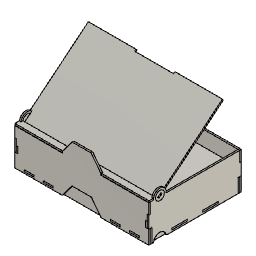
boite_h120_ep5_v2 (Autodesk Fusion 360 design; units mm, degrees)
Autodesk Fusion 360 part; units mm, degrees
note: some values were not read from the file. Set by a fixed rule: which sketch regions a step uses.
sketch "Esquisse1" plane through (0, 0, 0) normal (0, 1, 0) x (-1, 0, 0)
  line L0 (0, 0) -> (420, 0)
  line L1 (420, 0) -> (420, 120)
  line L2 (420, 120) -> (0, 120)
  line L3 (0, 120) -> (0, 0)
  line L4 (210, 0) -> (210, 120) construction
  line L5 (210, 40) -> (180, 40)
  line L6 (180, 40) -> (150, 0)
  line L7 (240, 40) -> (270, 0)
  line L8 (210, 40) -> (240, 40)
  line L9 (180, 160) -> (150, 120)
  line L10 (210, 160) -> (180, 160)
  line L11 (210, 160) -> (240, 160)
  line L12 (240, 160) -> (270, 120)
  line L13 (150, 5) -> (120, 5)
  line L14 (120, 5) -> (120, 10)
  line L15 (120, 10) -> (150, 10)
  line L16 (150, 10) -> (150, 5)
  line L17 (120, 5) -> (90, 5)
  line L18 (90, 5) -> (90, 10)
  line L19 (90, 10) -> (120, 10)
  line L20 (120, 10) -> (120, 5)
  line L21 (90, 5) -> (60, 5)
  line L22 (60, 5) -> (60, 10)
  line L23 (60, 10) -> (90, 10)
  line L24 (90, 10) -> (90, 5)
  line L25 (60, 5) -> (30, 5)
  line L26 (30, 5) -> (30, 10)
  line L27 (30, 10) -> (60, 10)
  line L28 (60, 10) -> (60, 5)
  line L29 (30, 5) -> (0, 5)
  line L30 (0, 5) -> (0, 10)
  line L31 (0, 10) -> (30, 10)
  line L32 (30, 10) -> (30, 5)
  line L33 (330, 5) -> (330, 10)
  line L34 (360, 10) -> (330, 10)
  line L35 (360, 5) -> (360, 10)
  line L36 (300, 10) -> (300, 5)
  line L37 (270, 5) -> (300, 5)
  line L38 (330, 5) -> (360, 5)
  line L39 (390, 5) -> (390, 10)
  line L40 (330, 10) -> (330, 5)
  line L41 (360, 10) -> (360, 5)
  line L42 (300, 5) -> (330, 5)
  line L43 (360, 5) -> (390, 5)
  line L44 (420, 5) -> (420, 10)
  line L45 (270, 10) -> (270, 5)
  line L46 (390, 10) -> (390, 5)
  line L47 (300, 10) -> (270, 10)
  line L48 (330, 10) -> (300, 10)
  line L49 (420, 10) -> (390, 10)
  line L50 (300, 5) -> (300, 10)
  line L51 (390, 10) -> (360, 10)
  line L52 (390, 5) -> (420, 5)
  line L53 (0, 5) -> (10, 5)
  line L54 (10, 5) -> (10, 43.3333)
  line L55 (10, 43.3333) -> (0, 43.3333)
  line L56 (0, 43.3333) -> (0, 5)
  line L57 (0, 43.3333) -> (10, 43.3333)
  line L58 (10, 81.6667) -> (0, 81.6667)
  line L59 (10, 43.3333) -> (10, 81.6667)
  line L60 (0, 81.6667) -> (10, 81.6667)
  line L61 (10, 120) -> (0, 120)
  line L62 (10, 81.6667) -> (10, 120)
  line L63 (410, 120) -> (420, 120)
  line L64 (420, 43.3333) -> (410, 43.3333)
  line L65 (410, 43.3333) -> (420, 43.3333)
  line L66 (410, 5) -> (410, 43.3333)
  line L67 (410, 81.6667) -> (410, 120)
  line L68 (420, 43.3333) -> (420, 5)
  line L69 (420, 5) -> (410, 5)
  line L70 (410, 81.6667) -> (420, 81.6667)
  line L71 (420, 81.6667) -> (410, 81.6667)
  line L72 (410, 43.3333) -> (410, 81.6667)
  line L73 (420, 5) -> (420, 10)
  line L74 (5, 43.3333) -> (5, 81.6667)
  line L75 (10, 62.5) -> (0, 62.5)
  line L76 (415, 81.6667) -> (415, 43.3333)
  line L77 (410, 62.5) -> (420, 62.5)
  line L78 (270, 120) -> (400, 120)
  line L79 (400, 120) -> (400, 115)
  line L80 (400, 115) -> (270, 115)
  line L81 (270, 115) -> (270, 120)
  line L82 (150, 120) -> (0, 120)
  line L83 (0, 120) -> (0, 115)
  line L84 (0, 115) -> (150, 115)
  line L85 (150, 115) -> (150, 120)
  line L86 (270, 115) -> (420, 115)
  line L87 (179.7, 40.6) -> (149.25, 0)
  line L88 (210, 40.6) -> (179.7, 40.6)
  line L89 (210, 40.6) -> (240.3, 40.6)
  line L90 (240.3, 40.6) -> (270.75, 0)
  point P0 (420, 120)
  dimension "d1" = 420
  dimension "d2" = 120
  dimension "d4" = 60
  dimension "d5" = 40
  dimension "d6" = 30
  dimension "d9" = 0
  dimension "d10" = 120
  dimension "d11" = 30
  dimension "d12" = 5
  dimension "d13" = 5
  dimension "d14" = 150
  dimension "d17" = -120
  dimension "d18" = 0
  dimension "d19" = 10
  dimension "d20" = 115
  dimension "d21" = 38.3333
  dimension "d24" = 0
  dimension "d25" = 76.6667
  dimension "d72" = 5
  dimension "d73" = 5
  constraint horizontal L0
  constraint vertical L1
  constraint horizontal L2
  constraint vertical L3
  constraint coincident L0.start L3.end
  constraint midpoint L0 L4.start
  constraint midpoint L2 L4.end
  constraint coincident L4 L5.start
  constraint perpendicular L4 L5
  constraint coincident L0 L6.end
  constraint symmetric L4 L5.start L8.start
  constraint symmetric L4 L5.end L7.start
  constraint symmetric L4 L6.end L7.end
  constraint horizontal L13
  constraint vertical L14
  constraint horizontal L15
  constraint vertical L16
  constraint coincident L6.end L16
  constraint symmetric L4 L13.start L37.start
  constraint symmetric L4 L13.end L36.end
  constraint symmetric L4 L14.end L36.start
  constraint symmetric L4 L15.end L45.start
  constraint symmetric L4 L17.end L33.start
  constraint symmetric L4 L18.end L33.end
  constraint symmetric L4 L21.end L35.start
  constraint symmetric L4 L22.end L34.start
  constraint symmetric L4 L25.end L39.start
  constraint symmetric L4 L26.end L39.end
  constraint symmetric L4 L29.end L44.start
  constraint symmetric L4 L30.end L44.end
  constraint horizontal L53
  constraint vertical L54
  constraint horizontal L55
  constraint vertical L56
  constraint symmetric L2.end L4 P0
  constraint symmetric L4 L53.end L66.start
  constraint symmetric L4 L54.end L64.end
  constraint symmetric L4 L55.end L64.start
  constraint symmetric L4 L58.start L67.start
  constraint symmetric L4 L58.end L70.end
  constraint symmetric L4 L61.start L63.start
  constraint symmetric L4 L2.end P0
  constraint midpoint L57 L74.start
  constraint midpoint L60 L74.end
  constraint midpoint L59 L75.start
  constraint coincident L3 L75.end
  constraint perpendicular L3 L75
  constraint midpoint L70 L76.start
  constraint midpoint L64 L76.end
  constraint midpoint L72 L77.start
  constraint coincident L1 L77.end
  constraint perpendicular L1 L77
  constraint horizontal L78
  constraint vertical L79
  constraint horizontal L80
  constraint vertical L81
  constraint horizontal L82
  constraint vertical L83
  constraint horizontal L84
  constraint vertical L85
  constraint coincident L1 L86.end
  constraint perpendicular L1 L86
  constraint coincident L0 L90.end
  constraint coincident L0 L87.end
  measures "d1" distance of L0.start L0.end
  measures "d2" distance of L0.start L2.end
  measures "d4" distance of L4.start L6.end
  measures "d5" distance of L0 L5
  measures "d6" distance of L5.start L5.end
  measures "d11" distance of L13.start L13.end
  measures "d12" distance of L13.start L15.end
  measures "d13" distance of L0 L13
  measures "d14" distance of L0.start L6.end
  measures "d19" distance of L54.end L55.end
  measures "d20" distance of L2 L29
  measures "d21" distance of L53 L55
  measures "d72" distance of L12.end L80.end
  measures "d73" distance of L9.end L84.end
extrude "Extrusion1" add sketch "Esquisse1" along normal blind 5 contours L0 L1 L2 L3 L13 L15 L16 L17 L19 L21 L23 L25 L27 L29 L31 L34 L37 L38 L42 L43 L45 L47 L48 L49 L51 L52 L53 L54 L59 L62 L66 L67 L69 L72 L80 L81 L84 L85 L86 L87 L88 L89 L90 | L3 L29 L30 L31 L53 L54 L56 | L3 L31 L54 L55 L56 L57 | L26 L29 L31 L32 L54 | L18 L21 L22 L23 L24 L28 | L3 L58 L60 L62 L84 | L58 L59 L60 L74 L75 | L1 L44 L49 L52 L66 L68 L69 L73 | L13 L14 L15 L16 L20 | L1 L49 L64 L65 L66 L68 | L39 L46 L49 L52 L66 | L33 L34 L35 L38 L40 L41 | L2 L9 L10 L11 L12 | L1 L67 L70 L71 L86 | L70 L71 L72 L76 L77 | L36 L37 L45 L47 L50 makes body 1
sketch "Esquisse2" plane through (0, 5, 0) normal (0, 1, 0) x (-1, 0, 0)
  line L0 (420, 0) -> (0, 0)
  line L1 (0, 0) -> (0, 62.5)
  line L2 (0, 62.5) -> (420, 62.5)
  line L3 (420, 62.5) -> (420, 0)
  line L4 (0, 10) -> (30, 10)
  line L5 (30, 10) -> (30, 5)
  line L6 (30, 5) -> (0, 5)
  line L7 (0, 5) -> (0, 10)
  line L8 (210, 62.5) -> (210, 0) construction
  line L9 (30, 10) -> (60, 10)
  line L10 (60, 5) -> (30, 5)
  line L11 (30, 5) -> (30, 10)
  line L12 (60, 10) -> (60, 5)
  line L13 (60, 10) -> (90, 10)
  line L14 (90, 5) -> (60, 5)
  line L15 (60, 5) -> (60, 10)
  line L16 (90, 10) -> (90, 5)
  line L17 (90, 10) -> (120, 10)
  line L18 (120, 5) -> (90, 5)
  line L19 (90, 5) -> (90, 10)
  line L20 (120, 10) -> (120, 5)
  line L21 (120, 10) -> (150, 10)
  line L22 (150, 5) -> (120, 5)
  line L23 (120, 5) -> (120, 10)
  line L24 (150, 10) -> (150, 5)
  line L25 (0, 62.5) -> (10, 62.5)
  line L26 (10, 62.5) -> (10, 43.3333)
  line L27 (10, 43.3333) -> (0, 43.3333)
  line L28 (0, 43.3333) -> (0, 62.5)
  line L29 (270, 10) -> (270, 5)
  line L30 (420, 62.5) -> (410, 62.5)
  line L31 (300, 10) -> (270, 10)
  line L32 (410, 43.3333) -> (420, 43.3333)
  line L33 (300, 5) -> (300, 10)
  line L34 (300, 5) -> (330, 5)
  line L35 (360, 5) -> (360, 10)
  line L36 (390, 5) -> (420, 5)
  line L37 (410, 62.5) -> (410, 43.3333)
  line L38 (270, 5) -> (300, 5)
  line L39 (420, 5) -> (420, 10)
  line L40 (330, 5) -> (330, 10)
  line L41 (390, 10) -> (360, 10)
  line L42 (420, 43.3333) -> (420, 62.5)
  line L43 (300, 10) -> (300, 5)
  line L44 (360, 10) -> (330, 10)
  line L45 (330, 10) -> (330, 5)
  line L46 (360, 10) -> (360, 5)
  line L47 (390, 5) -> (390, 10)
  line L48 (330, 10) -> (300, 10)
  line L49 (420, 0) -> (420, 62.5)
  line L50 (390, 10) -> (390, 5)
  line L51 (360, 5) -> (390, 5)
  line L52 (420, 10) -> (390, 10)
  line L53 (330, 5) -> (360, 5)
  line L54 (90, 10) -> (120, 10)
  line L55 (120, 10) -> (120, 5)
  line L56 (120, 5) -> (90, 5)
  line L57 (90, 5) -> (90, 10)
  line L58 (360, 10) -> (390, 10)
  line L59 (390, 10) -> (390, 5)
  line L60 (390, 5) -> (360, 5)
  line L61 (360, 5) -> (360, 10)
  line L62 (300, 10) -> (330, 10)
  line L63 (330, 10) -> (330, 5)
  line L64 (330, 5) -> (300, 5)
  line L65 (300, 5) -> (300, 10)
  line L66 (30, 10) -> (60, 10)
  line L67 (60, 10) -> (60, 5)
  line L68 (60, 5) -> (30, 5)
  line L69 (30, 5) -> (30, 10)
  line L70 (270.75, 0) -> (420, 0)
  line L71 (420, 0) -> (420, 43.3333)
  line L72 (420, 43.3333) -> (410, 43.3333)
  line L73 (410, 43.3333) -> (410, 62.5)
  line L74 (415, 81.6667) -> (420, 81.6667)
  line L75 (420, 81.6667) -> (420, 115)
  line L76 (270, 120) -> (240, 160)
  line L77 (240, 160) -> (180, 160)
  line L78 (180, 160) -> (150, 120)
  line L79 (0, 115) -> (0, 81.6667)
  line L80 (0, 81.6667) -> (5, 81.6667)
  line L81 (10, 62.5) -> (10, 43.3333)
  line L82 (10, 43.3333) -> (0, 43.3333)
  line L83 (0, 43.3333) -> (0, 0)
  line L84 (0, 0) -> (149.25, 0)
  line L85 (5, 81.6667) -> (5, 62.5)
  line L86 (5, 62.5) -> (10, 62.5)
  line L87 (410, 62.5) -> (415, 62.5)
  line L88 (415, 62.5) -> (415, 81.6667)
  line L89 (150, 120) -> (150, 115)
  line L90 (150, 115) -> (0, 115)
  line L91 (420, 115) -> (270, 115)
  line L92 (270, 115) -> (270, 120)
  line L93 (179.7, 40.6) -> (240.3, 40.6)
  line L94 (240.3, 40.6) -> (270.75, 0)
  line L95 (149.25, 0) -> (179.7, 40.6)
  point P0 (30, 0)
  point P1 (30, 0)
  point P2 (60, 0)
  point P3 (60, 0)
  point P4 (90, 0)
  point P5 (90, 0)
  point P6 (120, 0)
  point P7 (120, 0)
  point P8 (300, 0)
  point P9 (420, 0)
  point P10 (360, 0)
  point P11 (360, 0)
  point P12 (330, 0)
  point P13 (330, 0)
  point P14 (300, 0)
  point P15 (390, 0)
  point P16 (390, 0)
  dimension "d31" = 62.5
  dimension "d32" = 420
  dimension "d35" = 5
  dimension "d36" = 5
  dimension "d37" = 30
  dimension "d40" = 120
  dimension "d41" = 0
  dimension "d42" = 10
  dimension "d43" = 19.1667
  constraint horizontal L0
  constraint vertical L1
  constraint horizontal L2
  constraint vertical L3
  constraint horizontal L4
  constraint vertical L5
  constraint horizontal L6
  constraint vertical L7
  constraint coincident L1 L4.start
  constraint midpoint L2 L8.start
  constraint midpoint L0 L8.end
  constraint horizontal L25
  constraint vertical L26
  constraint horizontal L27
  constraint vertical L28
  constraint symmetric L0.end L8 P9
  constraint symmetric L1.end L8 L2.end
  constraint symmetric L4.start L8 L39.end
  constraint symmetric L4.end L8 L41.start
  constraint symmetric L5.end L8 L36.start
  constraint symmetric L6.end L8 L36.end
  constraint symmetric L8 L4.end L41.start
  constraint symmetric L8 L9.end L35.end
  constraint symmetric L8 L10.start L35.start
  constraint symmetric L8 L5.end L36.start
  constraint symmetric L8 P1 P16
  constraint symmetric L8 P1 P15
  constraint symmetric L8 L13.end L40.end
  constraint symmetric L8 L14.start L34.end
  constraint symmetric L8 P3 P11
  constraint symmetric L8 L17.end L31.start
  constraint symmetric L8 L18.start L33.start
  constraint symmetric L8 P5 P13
  constraint symmetric L8 L21.end L29.start
  constraint symmetric L8 L22.start L29.end
  constraint symmetric L8 P7 P14
  constraint symmetric L8 L25.end L30.end
  constraint symmetric L8 L26.end L32.start
  constraint symmetric L8 L27.end L32.end
  constraint collinear L1 L83
  measures "d31" distance of L0.end L1.end
  measures "d32" distance of P9 L0.end
  measures "d35" distance of L0 L6
  measures "d36" distance of L4 L6
  measures "d37" distance of L4.start L4.end
  measures "d42" distance of L1 L26
  measures "d43" distance of L25.end L26.end
extrude "Extrusion2" add sketch "Esquisse2" along normal blind 5 separate body contours L0 L1 L2 L3 L4 L6 L9 L10 L13 L14 L17 L18 L21 L22 L24 L26 L27 L29 L31 L32 L34 L36 L37 L38 L41 L44 L48 L49 L51 L52 L53 L54 L56 L58 L60 L62 L64 L66 L68 L70 L71 L72 L73 L81 L82 L83 L84 L93 L94 L95 | L0 L93 L94 L95 | L3 L36 L39 L47 L49 L50 L52 L59 L71 | L35 L40 L44 L45 L46 L53 L61 L63 | L1 L4 L5 L6 L7 L11 L69 L83 | L29 L31 L33 L38 L43 L65 | L12 L13 L14 L15 L16 L19 L57 L67 | L20 L21 L22 L23 L24 L55 makes body 2
sketch "Esquisse3" plane through (0, 0, 0) normal (1, 0, 0) x (0, 1, 0)
  line L0 (0, 0) -> (290, 0)
  line L1 (290, 0) -> (290, 120)
  line L2 (290, 120) -> (0, 120)
  line L3 (0, 120) -> (0, 0)
  line L4 (145, 120) -> (145, 0) construction
  line L5 (0, 120) -> (5, 120)
  line L6 (5, 120) -> (5, 81.6667)
  line L7 (5, 81.6667) -> (0, 81.6667)
  line L8 (0, 81.6667) -> (0, 120)
  line L9 (5, 43.3333) -> (0, 43.3333)
  line L10 (5, 81.6667) -> (5, 43.3333)
  line L11 (5, 5) -> (0, 5)
  line L12 (5, 43.3333) -> (5, 5)
  line L13 (0, 120) -> (10, 120)
  line L14 (10, 120) -> (10, 81.6667)
  line L15 (10, 81.6667) -> (0, 81.6667)
  line L16 (0, 81.6667) -> (0, 120)
  line L17 (10, 43.3333) -> (0, 43.3333)
  line L18 (0, 81.6667) -> (0, -38.3333)
  line L19 (0, 43.3333) -> (0, 81.6667)
  line L20 (0, 81.6667) -> (10, 81.6667)
  line L21 (10, 81.6667) -> (10, 43.3333)
  line L22 (10, 5) -> (0, 5)
  line L23 (0, 43.3333) -> (0, -76.6667)
  line L24 (0, 5) -> (0, 43.3333)
  line L25 (0, 43.3333) -> (10, 43.3333)
  line L26 (10, 43.3333) -> (10, 5)
  line L27 (15, 0) -> (0, 0)
  line L28 (0, 0) -> (0, 5)
  line L29 (275, 0) -> (290, 0)
  line L30 (280, 43.3333) -> (280, 5)
  line L31 (290, 81.6667) -> (290, 120)
  line L32 (290, 5) -> (290, 43.3333)
  line L33 (285, 81.6667) -> (290, 81.6667)
  line L34 (290, 120) -> (285, 120)
  line L35 (285, 120) -> (285, 81.6667)
  line L36 (285, 43.3333) -> (285, 0)
  line L37 (280, 81.6667) -> (280, 43.3333)
  line L38 (290, 43.3333) -> (290, 81.6667)
  line L39 (285, 43.3333) -> (290, 43.3333)
  line L40 (290, 81.6667) -> (280, 81.6667)
  line L41 (285, 81.6667) -> (285, 43.3333)
  line L42 (290, 43.3333) -> (280, 43.3333)
  line L43 (290, 0) -> (290, 5)
  line L44 (280, 43.3333) -> (290, 43.3333)
  line L45 (280, 81.6667) -> (290, 81.6667)
  line L46 (290, 120) -> (290, 0)
  line L47 (280, 5) -> (290, 5)
  line L48 (285, 5) -> (290, 5)
  line L49 (280, 120) -> (280, 81.6667)
  line L50 (290, 120) -> (280, 120)
  line L51 (290, 81.6667) -> (290, 120)
  line L52 (10, 100.8333) -> (0, 100.8333)
  line L53 (10, 62.5) -> (0, 62.5)
  line L54 (10, 24.1667) -> (0, 24.1667)
  line L55 (0, 120) -> (290, 120)
  line L56 (290, 120) -> (290, 115)
  line L57 (290, 115) -> (0, 115)
  line L58 (0, 115) -> (0, 120)
  line L59 (0, 117.5) -> (290, 117.5) construction
  circle A0 centre (35, 117.5) radius 20
  circle A1 centre (35, 117.5) radius 14
  line L60 (-12.3138, -2.5) -> (85, -2.5) construction
  circle A2 centre (35, -2.5) radius 20.3
  line L61 (72.5, 5) -> (217.5, 5)
  line L62 (217.5, 5) -> (217.5, 10)
  line L63 (217.5, 10) -> (72.5, 10)
  line L64 (72.5, 10) -> (72.5, 5)
  line L65 (0, 0) -> (10, 0)
  line L66 (10, 0) -> (10, 5)
  line L67 (10, 5) -> (0, 5)
  line L68 (0, 5) -> (0, 0)
  line L69 (290, 5) -> (280, 5)
  line L70 (280, 5) -> (280, 0)
  line L71 (280, 0) -> (290, 0)
  line L72 (290, 0) -> (290, 5)
  line L73 (120.8333, 10) -> (169.1667, 10)
  line L74 (169.1667, 10) -> (169.1667, 5)
  line L75 (169.1667, 5) -> (120.8333, 5)
  line L76 (120.8333, 5) -> (120.8333, 10)
  point P0 (290, 0)
  point P1 (5, 115)
  dimension "d45" = 290
  dimension "d46" = 120
  dimension "d47" = 5
  dimension "d48" = 38.3333
  dimension "d51" = 0
  dimension "d52" = -76.6667
  dimension "d53" = 38.3333
  dimension "d54" = 10
  dimension "d74" = 5
  dimension "d86" = 40
  dimension "d87" = 28
  dimension "d90" = 35
  dimension "d130" = 40.6
  dimension "d131" = 35
  dimension "d132" = 2.5
  dimension "d138" = 5
  dimension "d139" = 145
  dimension "d140" = 72.5
  dimension "d141" = 5
  dimension "d173" = 10
  dimension "d174" = 5
  dimension "d175" = 10
  dimension "d185" = 48.3333
  dimension "d186" = 48.3333
  constraint horizontal L0
  constraint vertical L1
  constraint horizontal L2
  constraint vertical L3
  constraint coincident L0.start L3.end
  constraint midpoint L2 L4.start
  constraint midpoint L0 L4.end
  constraint horizontal L5
  constraint vertical L6
  constraint horizontal L7
  constraint vertical L8
  constraint horizontal L13
  constraint vertical L14
  constraint horizontal L15
  constraint vertical L16
  constraint horizontal L27
  constraint vertical L28
  constraint coincident L0 L27.start
  constraint symmetric L0.start L4 L0.end
  constraint symmetric L0.start L4 P0
  constraint symmetric L2.end L4 L1.end
  constraint symmetric L4 L5.end L34.end
  constraint symmetric L4 L6.end L33.start
  constraint symmetric L4 L7.end L31.start
  constraint symmetric L4 L9.end L32.end
  constraint symmetric L4 L9.start L36.start
  constraint symmetric L4 L11.end L32.start
  constraint symmetric L4 L11.start L48.start
  constraint symmetric L4 L13.end L49.start
  constraint symmetric L4 L14.end L37.start
  constraint symmetric L4 L17.start L30.start
  constraint symmetric L4 L22.start L30.end
  constraint symmetric L4 L27.start L29.start
  constraint symmetric L4 L0.start P0
  constraint midpoint L14 L52.start
  constraint midpoint L16 L52.end
  constraint horizontal L55
  constraint vertical L56
  constraint horizontal L57
  constraint vertical L58
  constraint coincident L46 L56.end
  constraint midpoint L58 L59.start
  constraint midpoint L56 L59.end
  constraint coincident L59 A0.centre
  constraint concentric A0 A1
  constraint perpendicular L18 L60
  constraint coincident L60 A2.centre
  constraint horizontal L61
  constraint vertical L62
  constraint horizontal L63
  constraint vertical L64
  constraint horizontal L65
  constraint vertical L66
  constraint horizontal L67
  constraint vertical L68
  constraint horizontal L69
  constraint vertical L70
  constraint horizontal L71
  constraint vertical L72
  constraint coincident L29 L70.end
  constraint coincident L0 L36.end
  constraint coincident L48.start L36
  constraint horizontal L73
  constraint vertical L74
  constraint horizontal L75
  constraint vertical L76
  constraint coincident L61 L74.end
  constraint coincident L63 L73.start
  measures "d45" distance of L0.start P0
  measures "d46" distance of L0.start L2.end
  measures "d47" distance of L2.end L5.end
  measures "d48" distance of L2.end L7.end
  measures "d53" distance of L13.end L14.end
  measures "d54" distance of L14.end L7.end
  measures "d74" distance of L2 L57
  measures "d86" diameter of A0
  measures "d87" diameter of A1
  measures "d90" distance of L8 A0.centre
  measures "d130" diameter of A2
  measures "d131" distance of L23 A2.centre
  measures "d132" distance of L0 L60
  measures "d138" distance of L61.start L63.end
  measures "d139" distance of L62.end L63.end
  measures "d140" distance of L4 L62
  measures "d141" distance of L0 L61
  measures "d173" distance of L0.start L65.end
  measures "d174" distance of L11.end L0.start
  measures "d175" distance of L43 L70
  measures "d185" distance of L74 L76
  measures "d186" distance of L62 L74
extrude "Extrusion3" add sketch "Esquisse3" against normal blind 5 separate body contours L0 L14 L21 L26 L27 L29 L30 L37 L49 L57 A0 A2 L66 L70 | L3 L9 L10 L17 L18 L19 L25 L53 | L10 L17 L21 L25 L53 | L3 L7 L10 L15 L18 L19 L20 L53 | L10 L15 L20 L21 L53 | L6 L14 L15 L20 L52 | L37 L40 L41 L42 L44 L45 | L6 L14 L52 L57 | L1 L33 L38 L39 L40 L41 L42 L44 L45 L46 | L35 L40 L45 L49 L57 | L2 L55 L57 A0 A1 | L57 A0 A1 | L2 L55 L57 A0 A1 | L2 L55 A0 A1 | L61 L63 L73 L74 L75 L76 makes body 3
sketch "Esquisse4" plane through (-5, 0, 0) normal (-1, 0, 0) x (0, -1, 0)
  line L0 (-280, 0) -> (-55.1455, 0)
  line L1 (0, 0) -> (-290, 0)
  line L2 (-290, 0) -> (-290, 62.5)
  line L3 (-290, 62.5) -> (0, 62.5)
  line L4 (0, 62.5) -> (0, 0)
  line L5 (-290, 0) -> (-280, 0)
  line L6 (-280, 0) -> (-280, 43.3333)
  line L7 (-280, 43.3333) -> (-290, 43.3333)
  line L8 (-290, 43.3333) -> (-290, 0)
  line L9 (-145, 0) -> (-145, 115) construction
  line L10 (-72.5, 5) -> (-217.5, 5)
  line L11 (-217.5, 5) -> (-217.5, 10)
  line L12 (-217.5, 10) -> (-72.5, 10)
  line L13 (-72.5, 10) -> (-72.5, 5)
  line L14 (-72.5, 10) -> (-72.5, 5)
  line L15 (-169.1667, 5) -> (-217.5, 5)
  line L16 (-217.5, 5) -> (-217.5, 10)
  line L17 (-217.5, 10) -> (-169.1667, 10)
  circle A0 centre (-35, 117.5) radius 14
  line L18 (0, 43.3333) -> (0, 81.6667)
  line L19 (0, 81.6667) -> (-5, 81.6667)
  line L20 (-5, 81.6667) -> (-5, 115)
  line L21 (-5, 115) -> (-15.1569, 115)
  arc A1 (-15.1569, 115) -> (-54.8431, 115) centre (-35, 117.5) ccw
  line L22 (-54.8431, 115) -> (-285, 115)
  line L23 (-285, 115) -> (-285, 81.6667)
  line L24 (-285, 81.6667) -> (-290, 81.6667)
  line L25 (-290, 81.6667) -> (-290, 43.3333)
  line L26 (-290, 43.3333) -> (-280, 43.3333)
  arc A2 (-14.8545, 0) -> (-55.1455, 0) centre (-35, -2.5) ccw
  line L27 (-10, 43.3333) -> (0, 43.3333)
  line L28 (-280, 43.3333) -> (-280, 0)
  line L29 (-10, 0) -> (-10, 43.3333)
  line L30 (-120.8333, 10) -> (-169.1667, 10)
  line L31 (-169.1667, 10) -> (-169.1667, 5)
  line L32 (-169.1667, 5) -> (-120.8333, 5)
  line L33 (-120.8333, 5) -> (-120.8333, 10)
  line L34 (-169.1667, 10) -> (-169.1667, 5)
  line L35 (-120.8333, 5) -> (-120.8333, 10)
  line L36 (-120.8333, 10) -> (-72.5, 10)
  line L37 (-72.5, 5) -> (-120.8333, 5)
  line L38 (-14.8545, 0) -> (-10, 0)
  dimension "d62" = 62.5
  dimension "d63" = 10
  dimension "d64" = 43.3333
  dimension "d134" = 5
  dimension "d135" = 145
  dimension "d136" = 72.5
  dimension "d137" = 5
  dimension "d176" = 290
  dimension "d187" = 48.3333
  dimension "d188" = 48.3333
  constraint horizontal L1
  constraint vertical L2
  constraint horizontal L3
  constraint vertical L4
  constraint coincident L1.start L4.end
  constraint horizontal L5
  constraint vertical L6
  constraint horizontal L7
  constraint vertical L8
  constraint midpoint L1 L9.start
  constraint horizontal L10
  constraint vertical L11
  constraint horizontal L12
  constraint vertical L13
  constraint horizontal L30
  constraint vertical L31
  constraint horizontal L32
  constraint vertical L33
  constraint coincident L15 L31.end
  constraint coincident L12 L30.start
  measures "d62" distance of L1.end L2.end
  measures "d63" distance of L1.end L0.start
  measures "d64" distance of L5 L7
  measures "d134" distance of L10.end L11.end
  measures "d135" distance of L11.end L12.end
  measures "d136" distance of L9 L13
  measures "d137" distance of L1 L10
  measures "d176" distance of L2 L4
  measures "d187" distance of L30.start L17.end
  measures "d188" distance of L11 L31
extrude "Extrusion4" add sketch "Esquisse4" along normal blind 5 separate body contours L0 L1 L2 L3 L4 L6 L7 L18 L25 L26 A2 L27 L28 L29 L38 | L1 A2 | L10 L12 L30 L31 L32 L33 L34 L35 makes body 4
ref_plane "Plan de construction1" through (-210, 145, 80) normal (0, -1, 0) x (1, 0, 0)
mirror "Symétrie miroir2" about plane through (-210, 145, 80) normal (0, -1, 0) of bodies 1 2 makes body 5 at (-333.3333, 290, 80) makes body 6 at (-180, 280, 45)
ref_plane "Plan de construction2" through (-210, 0, 0) normal (1, 0, 0) x (0, 1, 0)
mirror "Symétrie miroir3" about plane through (-210, 0, 0) normal (1, 0, 0) of bodies 4 makes body 7
mirror "Symétrie miroir4" about plane through (-210, 0, 0) normal (1, 0, 0) of bodies 3 makes body 8
sketch "Esquisse5" plane through (0, 0, 0) normal (0, 0, 1) x (1, 0, 0)
  line L0 (59, -2.6937) -> (479, -2.6937)
  line L1 (479, -2.6937) -> (479, 287.3063)
  line L2 (479, 287.3063) -> (59, 287.3063)
  line L3 (59, 287.3063) -> (59, -2.6937)
  line L4 (208.2, -2.6937) -> (329.8, -2.6937)
  line L5 (329.8, -2.6937) -> (329.8, 2.6063)
  line L6 (329.8, 2.6063) -> (208.2, 2.6063)
  line L7 (208.2, 2.6063) -> (208.2, -2.6937)
  line L8 (479, 142.3063) -> (59, 142.3063) construction
  line L9 (479, 142.3063) -> (59, 142.3063) construction
  line L10 (208.2, 282.0063) -> (208.2, 287.3063)
  line L11 (329.8, 287.3063) -> (329.8, 282.0063)
  line L12 (208.2, 287.3063) -> (329.8, 287.3063)
  line L13 (329.8, 282.0063) -> (208.2, 282.0063)
  line L14 (479, 52.3063) -> (59, 52.3063) construction
  line L15 (479, 52.3063) -> (473.8, 52.3063)
  line L16 (473.8, 52.3063) -> (473.8, 0)
  line L17 (473.8, 0) -> (479, 0)
  line L18 (479, 0) -> (479, 52.3063)
  line L19 (269, -2.6937) -> (269, 287.3063) construction
  line L20 (479, 18.3063) -> (59, 18.3063)
  line L21 (64.2, 52.3063) -> (64.2, 0)
  line L22 (59, 52.3063) -> (64.2, 52.3063)
  line L23 (473.8, 25.6396) -> (479, 25.6396)
  line L24 (479, 25.6396) -> (479, 38.973)
  line L25 (479, 38.973) -> (473.8, 38.973)
  line L26 (473.8, 38.973) -> (473.8, 25.6396)
  line L27 (59, 38.973) -> (64.2, 38.973)
  line L28 (64.2, 38.973) -> (64.2, 25.6396)
  line L29 (64.2, 25.6396) -> (59, 25.6396)
  line L30 (59, 25.6396) -> (59, 38.973)
  line L31 (479, 17.0563) -> (59, 17.0563)
  line L32 (479, 52.3063) -> (473.8, 52.3063)
  line L33 (473.8, 11.0563) -> (479, 11.0563)
  line L34 (479, 11.0563) -> (479, 52.3063)
  line L35 (64.2, 11.0563) -> (59, 11.0563)
  line L36 (473.8, 32.3063) -> (479, 32.3063) construction
  dimension "d75" = 420
  dimension "d76" = 290
  dimension "d77" = 5.3
  dimension "d78" = 121.6
  dimension "d79" = 149.2
  dimension "d89" = 5.2
  dimension "d91" = 21
  dimension "d92" = 5.2
  dimension "d93" = 13.3333
  dimension "d94" = 13.3333
  dimension "d114" = 1.25
  dimension "d121" = 41.25
  dimension "d189" = 28.3333
  dimension "d190" = 35
  constraint horizontal L0
  constraint vertical L1
  constraint horizontal L2
  constraint vertical L3
  constraint horizontal L4
  constraint vertical L5
  constraint horizontal L6
  constraint vertical L7
  constraint coincident L0 L4.start
  constraint midpoint L1 L8.start
  constraint midpoint L3 L8.end
  constraint symmetric L4.start L8 L10.end
  constraint symmetric L4.end L8 L11.start
  constraint symmetric L5.end L8 L11.end
  constraint symmetric L6.end L8 L10.start
  constraint symmetric L9.start L8 L8.start
  constraint symmetric L9.end L8 L8.end
  constraint coincident L1 L14.start
  constraint coincident L3 L14.end
  constraint perpendicular L3 L14
  constraint horizontal L15
  constraint vertical L16
  constraint horizontal L17
  constraint vertical L18
  constraint midpoint L4 L19.start
  constraint midpoint L12 L19.end
  constraint coincident L18 L20.start
  constraint coincident L3 L20.end
  constraint perpendicular L3 L20
  constraint symmetric L14.start L19 L14.end
  constraint symmetric L15.end L19 L21.start
  constraint symmetric L16.end L19 L21.end
  constraint horizontal L23
  constraint vertical L24
  constraint horizontal L25
  constraint vertical L26
  constraint coincident L18 L24.end
  constraint coincident L16 L23.start
  constraint symmetric L19 L23.start L28.end
  constraint symmetric L19 L23.end L29.end
  constraint symmetric L19 L24.end L27.start
  constraint symmetric L19 L25.end L27.end
  constraint coincident L18 L31.start
  constraint coincident L3 L31.end
  constraint perpendicular L3 L31
  constraint horizontal L32
  constraint horizontal L33
  constraint vertical L34
  constraint symmetric L19 L33.start L35.start
  constraint symmetric L19 L33.end L35.end
  constraint midpoint L26 L36.start
  constraint midpoint L24 L36.end
  constraint coincident L16 L33.start
  measures "d75" distance of L0.start L0.end
  measures "d76" distance of L0.start L2.end
  measures "d77" distance of L4.start L6.end
  measures "d78" distance of L5.end L6.end
  measures "d79" distance of L3 L7
  measures "d89" distance of L14.start L15.end
  measures "d91" distance of L0 L20
  measures "d92" distance of L23.start L23.end
  measures "d93" distance of L23.start L25.end
  measures "d94" distance of L15 L25
  measures "d114" distance of L20 L31
  measures "d121" distance of L14.start L33.end
  measures "d189" distance of L0 L23
  measures "d190" distance of L0 L36
extrude "Extrusion5" add sketch "Esquisse5" along normal blind 5 separate body contours L3 L21 L27 L28 L29 L30 | L1 L2 L3 L10 L11 L13 L15 L16 L20 L21 L22 L26 L28 L32 | L1 L16 L18 L23 L24 L25 L26 L34 makes body 9
extrude "Extrusion7" add sketch "Esquisse5" along normal blind 5 separate body contours L0 L1 L3 L5 L6 L7 L16 L17 L21 L31 L35 | L1 L16 L17 L18 L33 makes body 10
copy_body "Corps->Comp1" bodies 9 removing the originals makes body 11 in component "Couvercle"
sketch "Esquisse6" plane through (0, 0, 0) normal (0, 0, 1) x (1, 0, 0)
  circle A0 centre (151.6667, -48.5) radius 13.9
  line L0 (145, -46) -> (158.3333, -46)
  line L1 (158.3333, -46) -> (158.3333, -51)
  line L2 (158.3333, -51) -> (145, -51)
  line L3 (145, -51) -> (145, -46)
  dimension "d95" = 27.8
  dimension "d96" = 13.3333
  dimension "d97" = 5
  dimension "d98" = 2.5
  dimension "d99" = 6.6667
  constraint horizontal L0
  constraint vertical L1
  constraint horizontal L2
  constraint vertical L3
  measures "d95" diameter of A0
  measures "d96" distance of L0.start L0.end
  measures "d97" distance of L0.start L2.end
  measures "d98" distance of A0.centre L2
  measures "d99" distance of A0.centre L3
extrude "Extrusion6" add sketch "Esquisse6" along normal blind 5 separate body makes body 12
copy_body "Corps->Comp2" bodies 12 removing the originals makes body 13 in component "pivot 2"
copy_body "Corps->Comp3" bodies 10 removing the originals makes body 14 in component "baguette-charniere"
sketch "Esquisse7" plane through (0, 0, 0) normal (0, 0, 1) x (1, 0, 0)
  line L0 (96, -5) -> (516, -5)
  line L1 (516, -5) -> (516, 285)
  line L2 (516, 285) -> (96, 285)
  line L3 (96, 285) -> (96, -5)
  line L4 (516, 140) -> (96, 140) construction
  line L5 (306, -5) -> (306, 285) construction
  line L6 (516, -5) -> (506, -5)
  line L7 (506, -5) -> (506, 67.5)
  line L8 (506, 67.5) -> (516, 67.5)
  line L9 (516, 67.5) -> (516, -5)
  line L10 (366, -5) -> (366, 285) construction
  line L11 (366, -5) -> (396, -5)
  line L12 (396, -5) -> (396, 5)
  line L13 (396, 5) -> (366, 5)
  line L14 (366, 5) -> (366, -5)
  line L15 (396, 5) -> (396, -5)
  line L16 (426, -5) -> (426, 5)
  line L17 (396, -5) -> (426, -5)
  line L18 (426, 5) -> (396, 5)
  line L19 (426, 5) -> (426, -5)
  line L20 (456, -5) -> (456, 5)
  line L21 (426, -5) -> (456, -5)
  line L22 (456, 5) -> (426, 5)
  line L23 (456, 5) -> (456, -5)
  line L24 (486, -5) -> (486, 5)
  line L25 (456, -5) -> (486, -5)
  line L26 (486, 5) -> (456, 5)
  line L27 (486, 5) -> (486, -5)
  line L28 (516, -5) -> (516, 5)
  line L29 (486, -5) -> (516, -5)
  line L30 (516, 5) -> (486, 5)
  line L31 (106, 67.5) -> (96, 67.5)
  line L32 (126, 5) -> (126, -5)
  line L33 (156, -5) -> (156, 5)
  line L34 (126, -5) -> (96, -5)
  line L35 (156, -5) -> (126, -5)
  line L36 (96, 67.5) -> (96, -5)
  line L37 (156, 5) -> (156, -5)
  line L38 (186, -5) -> (156, -5)
  line L39 (216, 5) -> (216, -5)
  line L40 (96, -5) -> (106, -5)
  line L41 (96, 5) -> (126, 5)
  line L42 (106, -5) -> (106, 67.5)
  line L43 (186, 5) -> (186, -5)
  line L44 (216, -5) -> (186, -5)
  line L45 (246, 5) -> (246, -5)
  line L46 (216, -5) -> (216, 5)
  line L47 (156, 5) -> (186, 5)
  line L48 (96, -5) -> (96, 5)
  line L49 (246, -5) -> (216, -5)
  line L50 (126, -5) -> (126, 5)
  line L51 (216, 5) -> (246, 5)
  line L52 (126, 5) -> (156, 5)
  line L53 (186, 5) -> (216, 5)
  line L54 (186, -5) -> (186, 5)
  line L55 (106, 212.5) -> (96, 212.5)
  line L56 (96, 285) -> (106, 285)
  line L57 (156, 275) -> (156, 285)
  line L58 (96, 285) -> (516, 285)
  line L59 (426, 275) -> (426, 285)
  line L60 (216, 275) -> (246, 275)
  line L61 (396, 285) -> (396, 275)
  line L62 (456, 275) -> (426, 275)
  line L63 (456, 285) -> (486, 285)
  line L64 (506, 212.5) -> (516, 212.5)
  line L65 (456, 275) -> (456, 285)
  line L66 (396, 275) -> (366, 275)
  line L67 (426, 285) -> (456, 285)
  line L68 (156, 275) -> (186, 275)
  line L69 (96, 275) -> (126, 275)
  line L70 (516, 275) -> (486, 275)
  line L71 (96, 212.5) -> (96, 285)
  line L72 (156, 285) -> (126, 285)
  line L73 (216, 285) -> (186, 285)
  line L74 (366, 275) -> (366, 285)
  line L75 (396, 285) -> (426, 285)
  line L76 (486, 275) -> (486, 285)
  line L77 (426, 275) -> (396, 275)
  line L78 (486, 285) -> (486, 275)
  line L79 (456, 285) -> (456, 275)
  line L80 (186, 275) -> (186, 285)
  line L81 (216, 285) -> (216, 275)
  line L82 (246, 275) -> (246, 285)
  line L83 (106, 285) -> (106, 212.5)
  line L84 (156, 285) -> (156, 275)
  line L85 (516, 212.5) -> (516, 285)
  line L86 (246, 285) -> (216, 285)
  line L87 (516, 285) -> (516, 275)
  line L88 (96, 285) -> (96, 275)
  line L89 (516, 285) -> (506, 285)
  line L90 (126, 285) -> (96, 285)
  line L91 (186, 275) -> (216, 275)
  line L92 (126, 285) -> (126, 275)
  line L93 (186, 285) -> (186, 275)
  line L94 (126, 275) -> (126, 285)
  line L95 (126, 275) -> (156, 275)
  line L96 (486, 285) -> (516, 285)
  line L97 (216, 275) -> (216, 285)
  line L98 (486, 275) -> (456, 275)
  line L99 (366, 285) -> (396, 285)
  line L100 (396, 275) -> (396, 285)
  line L101 (506, 285) -> (506, 212.5)
  line L102 (426, 285) -> (426, 275)
  line L103 (186, 285) -> (156, 285)
  line L104 (366, 5) -> (246, 5)
  line L105 (366, 275) -> (350, 275)
  line L106 (350, 275) -> (246, 275)
  line L107 (516, 164.1667) -> (506, 164.1667)
  line L108 (506, 164.1667) -> (506, 115.8333)
  line L109 (506, 115.8333) -> (516, 115.8333)
  line L110 (516, 115.8333) -> (516, 164.1667)
  line L111 (96, 164.1667) -> (106, 164.1667)
  line L112 (96, 140) -> (516, 140) construction
  line L113 (106, 115.8333) -> (96, 115.8333)
  line L114 (106, 164.1667) -> (106, 115.8333)
  point P0 (306, 285)
  dimension "d142" = 420
  dimension "d143" = 290
  dimension "d144" = 10
  dimension "d145" = 72.5
  dimension "d147" = 60
  dimension "d148" = 30
  dimension "d149" = 150
  dimension "d150" = 10
  dimension "d153" = 120
  dimension "d154" = 0
  dimension "d191" = 10
  dimension "d192" = 145
  dimension "d193" = 48.3333
  dimension "d194" = 24.1667
  constraint horizontal L0
  constraint vertical L1
  constraint horizontal L2
  constraint vertical L3
  constraint midpoint L1 L4.start
  constraint midpoint L3 L4.end
  constraint midpoint L0 L5.start
  constraint midpoint L2 P0
  constraint horizontal L6
  constraint vertical L7
  constraint horizontal L8
  constraint vertical L9
  constraint coincident L0 L10.start
  constraint coincident L2 L10.end
  constraint perpendicular L2 L10
  constraint horizontal L11
  constraint vertical L12
  constraint horizontal L13
  constraint vertical L14
  constraint symmetric L0.end L5 L0.start
  constraint symmetric L5 L6.end L40.end
  constraint symmetric L5 L7.end L31.start
  constraint symmetric L5 L8.end L31.end
  constraint symmetric L5 L10.start L45.end
  constraint symmetric L5 L11.end L39.end
  constraint symmetric L5 L12.end L39.start
  constraint symmetric L5 L13.end L45.start
  constraint symmetric L5 L16.start L38.start
  constraint symmetric L5 L16.end L43.start
  constraint symmetric L5 L20.start L33.start
  constraint symmetric L5 L20.end L33.end
  constraint symmetric L5 L24.start L32.end
  constraint symmetric L5 L24.end L32.start
  constraint symmetric L5 L0.end L0.start
  constraint symmetric L5 L28.end L41.start
  constraint symmetric L0.start L4 L2.end
  constraint symmetric L0.end L4 L1.end
  constraint symmetric L4 L5.start P0
  constraint symmetric L4 L6.end L89.end
  constraint symmetric L4 L7.end L64.start
  constraint symmetric L4 L8.end L64.end
  constraint symmetric L4 L10.start L10.end
  constraint symmetric L4 L11.end L61.start
  constraint symmetric L4 L12.end L61.end
  constraint symmetric L4 L13.end L66.end
  constraint symmetric L4 L16.start L59.end
  constraint symmetric L4 L16.end L59.start
  constraint symmetric L4 L20.start L63.start
  constraint symmetric L4 L20.end L62.start
  constraint symmetric L4 L24.start L63.end
  constraint symmetric L4 L24.end L70.end
  constraint symmetric L4 L0.end L1.end
  constraint symmetric L4 L28.end L70.start
  constraint symmetric L4 L32.start L69.end
  constraint symmetric L4 L43.start L68.end
  constraint symmetric L4 L38.start L73.end
  constraint symmetric L4 L39.end L73.start
  constraint symmetric L4 L39.start L60.start
  constraint symmetric L4 L0.start L2.end
  constraint symmetric L4 L33.start L57.end
  constraint symmetric L4 L32.end L72.end
  constraint symmetric L4 L45.start L60.end
  constraint symmetric L4 L41.start L69.start
  constraint symmetric L4 L40.end L56.end
  constraint symmetric L4 L45.end L82.end
  constraint symmetric L4 L31.start L55.start
  constraint symmetric L4 L31.end L55.end
  constraint symmetric L4 L33.end L57.start
  constraint perpendicular L74 L105
  constraint horizontal L107
  constraint vertical L108
  constraint horizontal L109
  constraint vertical L110
  constraint coincident L1 L107.start
  constraint symmetric L4.start L5 L4.end
  constraint symmetric L4.end L5 L4.start
  constraint symmetric L5 L107.start L111.start
  constraint symmetric L5 L107.end L111.end
  constraint symmetric L5 L108.end L113.start
  constraint symmetric L5 L109.end L113.end
  measures "d142" distance of L0.start L0.end
  measures "d143" distance of L0.start L2.end
  measures "d144" distance of L0.end L6.end
  measures "d145" distance of L0.end L8.end
  measures "d147" distance of L5 L10
  measures "d148" distance of L12.end L13.end
  measures "d149" distance of L1 L10
  measures "d150" distance of L10.start L13.end
  measures "d191" distance of L108.end L109.end
  measures "d192" distance of L8 L64
  measures "d193" distance of L107 L109
  measures "d194" distance of L4 L107
extrude "Extrusion8" add sketch "Esquisse7" along normal blind 5 separate body contours L0 L32 L33 L35 L37 L50 L52 | L1 L3 L7 L8 L13 L18 L22 L26 L30 L31 L41 L42 L47 L51 L52 L53 L55 L60 L62 L64 L66 L68 L69 L70 L77 L83 L91 L95 L98 L101 L104 L105 L106 L107 L108 L109 L111 L113 L114 | L0 L39 L43 L44 L46 L53 L54 | L0 L12 L15 L16 L17 L18 L19 | L2 L57 L58 L72 L84 L92 L94 L95 | L0 L20 L23 L24 L25 L26 L27 | L2 L58 L73 L80 L81 L91 L93 L97 | L2 L58 L59 L61 L75 L77 L100 L102 | L2 L58 L63 L65 L76 L78 L79 L98 makes body 15
copy_body "Corps->Comp4" bodies 15 removing the originals makes body 16 in component "fond"
copy_body "Corps->Comp5" bodies 7 removing the originals makes body 17 in component "cote-D-interieur"
copy_body "Corps->Comp7" bodies 6 removing the originals makes body 18 in component "face-interieur"
copy_body "Corps->Comp8" bodies 5 removing the originals makes body 19 in component "face-exterieur"
copy_body "Corps->Comp9" bodies 4 removing the originals makes body 20 in component "cote-G-interieur"
copy_body "Corps->Comp11" bodies 2 removing the originals makes body 21 in component "arriere-interieur"
copy_body "Corps->Comp12" bodies 1 removing the originals makes body 22 in component "arriere_exterieur"
copy_body "Corps->Comp15" bodies 8 removing the originals makes body 23 in component "cote-D-exterieur"
copy_body "Corps->Comp16" bodies 3 removing the originals makes body 24 in component "cote-G-exterieur"
sketch "Esquisse8" plane through (0, 0, 0) normal (0, 0, 1) x (1, 0, 0)
  line L0 (109.7851, 32.8439) -> (513.7851, 32.8439)
  line L1 (515.7851, 34.8439) -> (515.7851, 308.8439)
  line L2 (513.7851, 310.8439) -> (109.7851, 310.8439)
  line L3 (107.7851, 308.8439) -> (107.7851, 34.8439)
  circle A0 centre (311.7851, 270.8439) radius 17.5
  arc A1 (513.7851, 32.8439) -> (515.7851, 34.8439) centre (513.7851, 34.8439) ccw
  arc A2 (107.7851, 34.8439) -> (109.7851, 32.8439) centre (109.7851, 34.8439) ccw
  arc A3 (109.7851, 310.8439) -> (107.7851, 308.8439) centre (109.7851, 308.8439) ccw
  arc A4 (515.7851, 308.8439) -> (513.7851, 310.8439) centre (513.7851, 308.8439) ccw
  point P0 (107.7851, 32.8439)
  point P1 (515.7851, 32.8439)
  point P2 (107.7851, 310.8439)
  dimension "d161" = 408
  dimension "d162" = 278
  dimension "d163" = 35
  dimension "d164" = 40
  dimension "d165" = 204
  dimension "d168" = 2
  constraint horizontal L0
  constraint vertical L1
  constraint horizontal L2
  constraint vertical L3
  constraint coincident P1 L1
  constraint coincident P1 L0
  constraint tangent L1 A1
  constraint tangent L0 A1
  constraint coincident P0 L0
  constraint coincident P0 L3
  constraint tangent L0 A2
  constraint tangent L3 A2
  constraint equal A1 A2
  constraint coincident P2 L2
  constraint coincident P2 L3
  constraint tangent L2 A3
  constraint tangent L3 A3
  constraint equal A1 A3
  constraint tangent L1 A4
  constraint tangent L2 A4
  constraint equal A1 A4
  measures "d161" distance of P0 P1
  measures "d162" distance of P0 P2
  measures "d163" diameter of A0
  measures "d164" distance of L2 A0.centre
  measures "d165" distance of L3 A0.centre
  measures "d168" radius of A1
extrude "Extrusion9" add sketch "Esquisse8" along normal blind 5 separate body makes body 25
copy_body "Corps->Comp13" bodies 25 removing the originals makes body 26 in component "Couvercle median"
component "Couvercle" placed x (1, 0, 0) y (0, 1, 0) z (0, 0, 1) at (-479, 2.6937, 115)
component "pivot 2" placed x (0, -1, 0) y (0, 0, 1) z (-1, 0, 0) at (-415, 186.6667, 166)
component "pivot 2" placed x (0, 1, 0) y (0, 0, 1) z (1, 0, 0) at (-5, -116.6667, 166)
component "baguette-charniere" placed x (1, 0, 0) y (0, 1, 0) z (0, 0, 1) at (-479, 3.6006, 115)
component "fond" placed x (1, 0, 0) y (0, 1, 0) z (0, 0, 1) at (-516, 5, 5)
component "cote-D-interieur" placed x (1, 0, 0) y (0, 1, 0) z (0, 0, 1) at (0, 0, 0)
component "face-interieur" placed x (1, 0, 0) y (0, 1, 0) z (0, 0, 1) at (0, 0, 0)
component "face-exterieur" placed x (1, 0, 0) y (0, 1, 0) z (0, 0, 1) at (0, 0, 0)
component "cote-G-interieur" placed x (1, 0, 0) y (0, 1, 0) z (0, 0, 1) at (0, 0, 0)
component "arriere-interieur" placed x (1, 0, 0) y (0, 1, 0) z (0, 0, 1) at (0, 0, 0)
component "arriere_exterieur" placed x (1, 0, 0) y (0, 1, 0) z (0, 0, 1) at (0, 0, 0)
component "cote-D-exterieur" placed x (1, 0, 0) y (0, 1, 0) z (0, 0, 1) at (0, 0, 0)
component "cote-G-exterieur" placed x (1, 0, 0) y (0, 1, 0) z (0, 0, 1) at (0, 0, 0)
component "Couvercle median" placed x (1, 0, 0) y (0, 1, 0) z (0, 0, 1) at (-521.7851, -25.8439, 62.5)
equation "d1 = Lbx"
equation "d2 = Hbx"
equation "d10 = d2"
equation "d11 = d14 / 5"
equation "d12 = Ep_fond"
equation "d17 = -d14 + d11"
equation "d19 = 2 * Ep_bois"
equation "d21 = d20 / 3"
equation "d25 = d20 - d21"
equation "d26 = Ep_bois"
equation "Lbx = 420 mm" comment "Largeur de la boite"
equation "Hbx = 120 mm" comment "Hauteur externe de la boite"
equation "Ep_fond = 5 mm" comment "Eppaisseur du fond"
equation "d31 = ( ( Hbx + 5 mm ) / 2 )"
equation "d32 = Lbx"
equation "d33 = Ep_bois"
equation "d36 = Ep_fond"
equation "d37 = ( ( Lbx / 2 ) - d4 ) / 5"
equation "d40 = ( ( Lbx / 2 ) - d4 ) - d37"
equation "d42 = 2 * Ep_bois"
equation "d43 = ( ( Hbx - 5 mm ) / 2 ) / 3"
equation "Pbx = 290 mm" comment "Profondeur de la boite en extérieur"
equation "d45 = Pbx"
equation "d46 = Hbx"
equation "d47 = Ep_bois"
equation "d48 = ( Hbx - 5 mm ) / 3"
equation "d52 = -Hbx + 5 mm + d48"
equation "d53 = d48"
equation "d54 = Ep_bois * 2"
equation "d56 = -Ep_bois"
equation "d58 = -Pbx / 2"
equation "d62 = ( Hbx + 5 mm ) / 2"
equation "d63 = Ep_bois * 2"
equation "d64 = ( ( Hbx - 5 mm ) / 3 ) + 5 mm"
equation "d65 = Ep_bois"
equation "d69 = -Lbx / 2"
equation "d72 = Ep_bois"
equation "d73 = Ep_bois"
equation "d74 = Ep_bois"
equation "d75 = Lbx"
equation "d76 = Pbx"
equation "d77 = Ep_bois + 0.3 mm"
equation "d79 = ( d75 - d78 ) / 2"
equation "d80 = Ep_bois"
equation "d89 = Ep_bois + 0.2 mm"
equation "d90 = ( d86 / 2 ) + d54 + 5 mm"
equation "d93 = d86 / 3"
equation "d94 = d93"
equation "d96 = d86 / 3"
equation "d97 = Ep_bois"
equation "d98 = d97 / 2"
equation "d99 = d96 / 2"
equation "d114 = Ep_bois / 4"
equation "d115 = Ep_bois"
equation "d121 = d86 + ( Ep_bois / 4 )"
equation "d130 = d86 + 0.6 mm"
equation "d131 = d90"
equation "d132 = Ep_bois / 2"
equation "d134 = Ep_fond"
equation "d135 = Pbx / 2"
equation "d136 = d135 / 2"
equation "d138 = Ep_fond"
equation "d139 = Pbx / 2"
equation "d140 = d139 / 2"
equation "d142 = Lbx"
equation "d143 = Pbx"
equation "d144 = Ep_bois * 2"
equation "d145 = Pbx / 4"
equation "d147 = d4"
equation "d148 = d149 / 5"
equation "d150 = d144"
equation "d153 = -d148 + d149"
equation "d155 = Ep_fond"
equation "d161 = Lbx - ( 2 * Ep_bois ) - 2 mm"
equation "d162 = Pbx - ( 2 * Ep_bois ) - 2 mm"
equation "d165 = d161 / 2"
equation "d166 = Ep_bois"
equation "d175 = Ep_bois * 2"
equation "d176 = Pbx"
equation "Ep_bois = 5 mm" comment "Eppaisseur de bois"
equation "d185 = d139 / 3"
equation "d186 = d185"
equation "d187 = d135 / 3"
equation "d188 = d187"
equation "d189 = d90 - ( d93 / 2 )"
equation "d191 = d144"
equation "d193 = d192 / 3"
equation "d194 = d193 / 2"
named bodies: "cote-G-exterieur", "face-exterieur", "face-interieur", "cote-D-exterieur"
